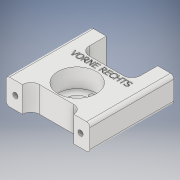
# Autodesk Inventor part: Motorhalterung leicht VR
Saved by Autodesk Inventor 2018 (Build 220112000, 112)
## iProperties
Created: 2019-03-03
Part Number: Motorhalterung leicht VR
Material: ABS-Kunststoff
Document SubType Name: Modeling
Designer: RedBots
Density: 0.513105 g/cm^3
Appearance: Weiß
Mass: 11 g
Surface Area: 84.958 cm^2
Volume: 21.4381 cm^3
Author: RedBots
Autodesk Inventor part; units mm, degrees
ref_plane "YZ Plane" through (0, 0, 0) normal (1, 0, 0) x (0, 1, 0)
ref_plane "XZ Plane" through (0, 0, 0) normal (0, 1, 0) x (-1, 0, 0)
ref_plane "XY Plane" through (0, 0, 0) normal (0, 0, 1) x (1, 0, 0)
sketch "Skizze2" plane through (0, 0, 0) normal (0, 0, 1) x (1, 0, 0)
  line L0 (0, 0) -> (49, 0)
  line L1 (0, 0) -> (49, 0) construction
  line L2 (49, 0) -> (49, 49)
  line L3 (49, 49) -> (0, 49)
  line L4 (0, 49) -> (0, 0)
  dimension "d16" = 49
  dimension "d18" = 49
  constraints: 10 end point, 2 equal length, 2 horizontal, 2 perpendicular
  measures "d16" distance of L0.start L0.end
  measures "d18" distance of L0.end L2.end
extrude "Extrusion1" add sketch "Skizze2" along normal blind 15
sketch "Skizze3" plane through (0, 0, 15) normal (0, 0, 1) x (1, 0, 0)
  circle A0 centre (24.5, 17) radius 11.25
  line L0 (0, 49) -> (0, 0) construction
  line L1 (0, 17) -> (49, 17) construction
  line L2 (49, 0) -> (49, 49) construction
  line L3 (0, 0) -> (49, 0) construction
  dimension "d72" = 22.5
  dimension "d73" = 17
  constraints: 2 end point, 2 point on line, 1 centre point, 1 coincident, 1 horizontal, 1 midpoint
  measures "d72" diameter of A0
  measures "d73" distance between parallel lines of L3 L1
extrude "Extrusion2" cut sketch "Skizze3" against normal blind 11
sketch "Skizze4" plane through (24.5, 17, 4) normal (0, 0, 1) x (1, 0, 0)
  circle A0 centre (7.3612, -4.25) radius 1.5
  circle A1 centre (0, 8.5) radius 1.5
  circle A2 centre (-7.3612, -4.25) radius 1.5
  line L0 (0, 0) -> (0, 8.5) construction
  line L1 (-24.5, -17) -> (24.5, -17) construction
  circle A3 centre (0, 0) radius 11.25 construction
  line L2 (0, -17) -> (0, 0) construction
  line L3 (0, 0) -> (7.3612, -4.25) construction
  line L4 (0, 0) -> (-7.3612, -4.25) construction
  circle A4 centre (0, 0) radius 6.5
  dimension "d37" = 3
  dimension "d42" = 3
  dimension "d43" = 3
  dimension "d90" = 8.5
  dimension "d91" = 120
  dimension "d92" = 120
  dimension "d93" = 13
  constraints: 8 end point, 4 centre point, 4 coincident, 2 equal length, 2 vertical, 1 midpoint
  measures "d37" diameter of A0
  measures "d42" diameter of A1
  measures "d43" diameter of A2
  measures "d90" distance of L0.start L0.end
  measures "d91" angle of L3 L0
  measures "d92" angle of L0 L4
  measures "d93" diameter of A4
extrude "Extrusion3" cut sketch "Skizze4" against normal up to next
sketch "Skizze9" plane through (0, 49, 0) normal (0, 1, 0) x (1, 0, 0)
  line L0 (24.5, -7.5) -> (43.5, -7.5) construction
  circle A0 centre (5.5, -7.5) radius 1.5
  circle A1 centre (43.5, -7.5) radius 1.5
  line L1 (0, -15) -> (49, -15) construction
  line L2 (24.5, -15) -> (24.5, 0) construction
  line L3 (49, 0) -> (0, 0) construction
  line L4 (5.5, -7.5) -> (24.5, -7.5) construction
  dimension "d58" = 3
  dimension "d89" = 19
  constraints: 7 end point, 3 midpoint, 2 centre point, 2 collinear, 1 coincident, 1 equal radius, 1 horizontal, 1 vertical
  measures "d58" diameter of A0
  measures "d89" distance of L0.start L0.end
extrude "Extrusion6" cut sketch "Skizze9" against normal blind 56
sketch "Skizze12" plane through (0, 0, 0) normal (0, 0, -1) x (-1, 0, 0)
  circle A0 centre (-24.5, 25.5) radius 1.5 projected
  circle A1 centre (-24.5, 25.5) radius 3
  circle A2 centre (-17.1388, 12.75) radius 1.5 projected
  circle A3 centre (-17.1388, 12.75) radius 3
  circle A4 centre (-31.8612, 12.75) radius 1.5 projected
  circle A5 centre (-31.8612, 12.75) radius 3
  point P0 (0, 0)
  dimension "d80" = 6
  dimension "d81" = 6
  dimension "d82" = 6
  constraints: 3 centre point, 3 coincident
  measures "d80" diameter of A1
  measures "d81" diameter of A3
  measures "d82" diameter of A5
extrude "Extrusion8" cut sketch "Skizze12" against normal blind 0.16
chamfer "Fase3" distance 1.5 angle 45 3 edges at (23, 25.5, 0.16) (30.3612, 12.75, 0.16) (15.6388, 12.75, 0.16)
fillet "Rundung2" radius 0.5 3 edges at (23, 25.5, 1.66) (30.3612, 12.75, 1.66) (15.6388, 12.75, 1.66)
sketch "Skizze14" plane through (0, 0, 0) normal (0, 0, -1) x (-1, 0, 0)
  line L0 (-39.5, 49) -> (-9.5, 49)
  line L1 (-9.5, 49) -> (-9.5, 34)
  line L2 (-9.5, 34) -> (-39.5, 34)
  line L3 (-39.5, 34) -> (-39.5, 49)
  line L4 (-49, 49) -> (0, 49) projected
  line L5 (-49, 0) -> (-49, 49) construction
  line L6 (0, 49) -> (0, 0) construction
  line L7 (-39.5, 0) -> (-9.5, 0)
  line L8 (-9.5, 0) -> (-9.5, 5)
  line L9 (-9.5, 5) -> (-39.5, 5)
  line L10 (-39.5, 5) -> (-39.5, 0)
  line L11 (0, 0) -> (-49, 0) projected
  point P0 (-24.5, 49)
  point P1 (-24.5, 0)
  point P2 (-24.5, 0)
  dimension "d95" = 15
  dimension "d96" = 30
  dimension "d101" = 5
  constraints: 16 end point, 6 midpoint, 3 horizontal, 3 parallel, 2 vertical, 1 perpendicular
  measures "d95" distance of L0.end L1.end
  measures "d96" distance between parallel lines of L1 L3
  measures "d101" distance of L7.end L9.start
extrude "Extrusion9" cut sketch "Skizze14" against normal up to next
fillet "Rundung3" radius 5 4 edges at (39.5, 34, 7.5) (9.5, 34, 7.5) (39.5, 5, 7.5) (9.5, 5, 7.5)
fillet "Rundung4" radius 2 4 edges at (49, 24.5, 15) (49, 24.5, 0) (0, 24.5, 0) (0, 24.5, 15)
sketch "Skizze15" plane through (0, 0, 15) normal (0, 0, 1) x (1, 0, 0)
  line L0 (14.5, 34) -> (34.5, 34) construction
  line L1 (24.5, 34) -> (24.5, 28.25) construction
  circle A0 centre (24.5, 17) radius 11.25 construction
  line L2 (10.3922, 32.875) -> (9.1868, 29.375)
  line L3 (9.1868, 29.375) -> (8.6848, 29.375)
  line L4 (8.6848, 29.375) -> (7.4793, 32.875)
  line L5 (7.4793, 32.875) -> (7.9785, 32.875)
  line L6 (7.9785, 32.875) -> (8.9485, 29.9678)
  line L7 (8.9485, 29.9678) -> (9.9186, 32.875)
  line L8 (9.9186, 32.875) -> (10.3922, 32.875)
  spline S0 degree 2 poles (13.203, 32.4751) (13.4015, 32.2425) (13.6228, 31.5618) (13.6228, 31.125) knots 0 0 0 1 2 2 2
  spline S1 degree 2 poles (13.6228, 31.125) (13.6228, 30.6996) (13.4072, 30.0103) (13.203, 29.7778) knots 0 0 0 1 2 2 2
  spline S2 degree 2 poles (13.203, 29.7778) (12.9874, 29.5338) (12.4173, 29.3013) (12.0741, 29.3013) knots 0 0 0 1 2 2 2
  spline S3 degree 2 poles (12.0741, 29.3013) (11.7196, 29.3013) (11.1523, 29.5423) (10.9453, 29.7778) knots 0 0 0 1 2 2 2
  spline S4 degree 2 poles (10.9453, 29.7778) (10.7439, 30.0103) (10.5284, 30.6939) (10.5284, 31.125) knots 0 0 0 1 2 2 2
  spline S5 degree 2 poles (10.5284, 31.125) (10.5284, 31.5646) (10.7468, 32.234) (10.9481, 32.4751) knots 0 0 0 1 2 2 2
  spline S6 degree 2 poles (10.9481, 32.4751) (11.1523, 32.7077) (11.7224, 32.9487) (12.0741, 32.9487) knots 0 0 0 1 2 2 2
  spline S7 degree 2 poles (12.0741, 32.9487) (12.4315, 32.9487) (13.0045, 32.6991) (13.203, 32.4751) knots 0 0 0 1 2 2 2
  spline S8 degree 2 poles (13.1378, 31.125) (13.1378, 31.471) (12.9874, 32.0071) (12.8513, 32.1829) knots 0 0 0 1 2 2 2
  spline S9 degree 2 poles (12.8513, 32.1829) (12.7123, 32.3645) (12.3209, 32.546) (12.077, 32.546) knots 0 0 0 1 2 2 2
  spline S10 degree 2 poles (12.077, 32.546) (11.8246, 32.546) (11.4445, 32.3701) (11.2998, 32.1829) knots 0 0 0 1 2 2 2
  spline S11 degree 2 poles (11.2998, 32.1829) (11.1609, 32.0043) (11.0134, 31.4654) (11.0134, 31.125) knots 0 0 0 1 2 2 2
  spline S12 degree 2 poles (11.0134, 31.125) (11.0134, 30.4358) (11.592, 29.704) (12.077, 29.704) knots 0 0 0 1 2 2 2
  spline S13 degree 2 poles (12.077, 29.704) (12.562, 29.704) (13.1378, 30.4358) (13.1378, 31.125) knots 0 0 0 1 2 2 2
  line L9 (16.842, 29.375) -> (16.2378, 29.375)
  line L10 (16.2378, 29.375) -> (15.1317, 30.7676)
  line L11 (15.1317, 30.7676) -> (14.5985, 30.7676)
  line L12 (14.5985, 30.7676) -> (14.5985, 29.375)
  line L13 (14.5985, 29.375) -> (14.1333, 29.375)
  line L14 (14.1333, 29.375) -> (14.1333, 32.875)
  line L15 (14.1333, 32.875) -> (15.0353, 32.875)
  spline S14 degree 2 poles (15.0353, 32.875) (15.3359, 32.875) (15.7415, 32.8098) (15.9259, 32.6906) knots 0 0 0 1 2 2 2
  spline S15 degree 2 poles (15.9259, 32.6906) (16.1102, 32.5715) (16.3229, 32.2) (16.3229, 31.9248) knots 0 0 0 1 2 2 2
  spline S16 degree 2 poles (16.3229, 31.9248) (16.3229, 31.5419) (15.9315, 31.0229) (15.5968, 30.8981) knots 0 0 0 1 2 2 2
  line L16 (15.5968, 30.8981) -> (16.842, 29.375)
  spline S17 degree 2 poles (15.8379, 31.888) (15.8379, 32.0411) (15.7301, 32.2765) (15.6167, 32.3531) knots 0 0 0 1 2 2 2
  spline S18 degree 2 poles (15.6167, 32.3531) (15.5174, 32.4184) (15.2536, 32.4722) (15.0608, 32.4722) knots 0 0 0 1 2 2 2
  line L17 (15.0608, 32.4722) -> (14.5985, 32.4722)
  line L18 (14.5985, 32.4722) -> (14.5985, 31.1562)
  line L19 (14.5985, 31.1562) -> (15.0069, 31.1562)
  spline S19 degree 2 poles (15.0069, 31.1562) (15.2083, 31.1562) (15.5288, 31.2271) (15.6394, 31.3377) knots 0 0 0 1 2 2 2
  spline S20 degree 2 poles (15.6394, 31.3377) (15.7415, 31.4342) (15.8379, 31.7064) (15.8379, 31.888) knots 0 0 0 1 2 2 2
  line L20 (19.6244, 29.375) -> (19.1025, 29.375)
  line L21 (19.1025, 29.375) -> (17.5539, 32.3928)
  line L22 (17.5539, 32.3928) -> (17.5539, 29.375)
  line L23 (17.5539, 29.375) -> (17.1199, 29.375)
  line L24 (17.1199, 29.375) -> (17.1199, 32.875)
  line L25 (17.1199, 32.875) -> (17.7808, 32.875)
  line L26 (17.7808, 32.875) -> (19.1904, 30.1039)
  line L27 (19.1904, 30.1039) -> (19.1904, 32.875)
  line L28 (19.1904, 32.875) -> (19.6244, 32.875)
  line L29 (19.6244, 32.875) -> (19.6244, 29.375)
  line L30 (20.3335, 29.375) -> (20.3335, 32.875)
  line L31 (20.3335, 32.875) -> (22.5231, 32.875)
  line L32 (22.5231, 32.875) -> (22.5231, 32.4609)
  line L33 (22.5231, 32.4609) -> (20.7986, 32.4609)
  line L34 (20.7986, 32.4609) -> (20.7986, 31.5022)
  line L35 (20.7986, 31.5022) -> (22.4068, 31.5022)
  line L36 (22.4068, 31.5022) -> (22.4068, 31.0881)
  line L37 (22.4068, 31.0881) -> (20.7986, 31.0881)
  line L38 (20.7986, 31.0881) -> (20.7986, 29.7891)
  line L39 (20.7986, 29.7891) -> (22.5231, 29.7891)
  line L40 (22.5231, 29.7891) -> (22.5231, 29.375)
  line L41 (22.5231, 29.375) -> (20.3335, 29.375)
  line L42 (27.2455, 29.375) -> (26.6414, 29.375)
  line L43 (26.6414, 29.375) -> (25.5353, 30.7676)
  line L44 (25.5353, 30.7676) -> (25.002, 30.7676)
  line L45 (25.002, 30.7676) -> (25.002, 29.375)
  line L46 (25.002, 29.375) -> (24.5369, 29.375)
  line L47 (24.5369, 29.375) -> (24.5369, 32.875)
  line L48 (24.5369, 32.875) -> (25.4388, 32.875)
  spline S21 degree 2 poles (25.4388, 32.875) (25.7395, 32.875) (26.1451, 32.8098) (26.3294, 32.6906) knots 0 0 0 1 2 2 2
  spline S22 degree 2 poles (26.3294, 32.6906) (26.5138, 32.5715) (26.7265, 32.2) (26.7265, 31.9248) knots 0 0 0 1 2 2 2
  spline S23 degree 2 poles (26.7265, 31.9248) (26.7265, 31.5419) (26.3351, 31.0229) (26.0004, 30.8981) knots 0 0 0 1 2 2 2
  line L49 (26.0004, 30.8981) -> (27.2455, 29.375)
  spline S24 degree 2 poles (26.2415, 31.888) (26.2415, 32.0411) (26.1337, 32.2765) (26.0203, 32.3531) knots 0 0 0 1 2 2 2
  spline S25 degree 2 poles (26.0203, 32.3531) (25.921, 32.4184) (25.6572, 32.4722) (25.4643, 32.4722) knots 0 0 0 1 2 2 2
  line L50 (25.4643, 32.4722) -> (25.002, 32.4722)
  line L51 (25.002, 32.4722) -> (25.002, 31.1562)
  line L52 (25.002, 31.1562) -> (25.4105, 31.1562)
  spline S26 degree 2 poles (25.4105, 31.1562) (25.6118, 31.1562) (25.9323, 31.2271) (26.0429, 31.3377) knots 0 0 0 1 2 2 2
  spline S27 degree 2 poles (26.0429, 31.3377) (26.1451, 31.4342) (26.2415, 31.7064) (26.2415, 31.888) knots 0 0 0 1 2 2 2
  line L53 (27.5235, 29.375) -> (27.5235, 32.875)
  line L54 (27.5235, 32.875) -> (29.7131, 32.875)
  line L55 (29.7131, 32.875) -> (29.7131, 32.4609)
  line L56 (29.7131, 32.4609) -> (27.9887, 32.4609)
  line L57 (27.9887, 32.4609) -> (27.9887, 31.5022)
  line L58 (27.9887, 31.5022) -> (29.5968, 31.5022)
  line L59 (29.5968, 31.5022) -> (29.5968, 31.0881)
  line L60 (29.5968, 31.0881) -> (27.9887, 31.0881)
  line L61 (27.9887, 31.0881) -> (27.9887, 29.7891)
  line L62 (27.9887, 29.7891) -> (29.7131, 29.7891)
  line L63 (29.7131, 29.7891) -> (29.7131, 29.375)
  line L64 (29.7131, 29.375) -> (27.5235, 29.375)
  spline S28 degree 2 poles (31.5908, 29.3126) (31.2504, 29.3126) (30.6746, 29.5423) (30.4647, 29.7721) knots 0 0 0 1 2 2 2
  spline S29 degree 2 poles (30.4647, 29.7721) (30.2549, 29.999) (30.0251, 30.6797) (30.0251, 31.1222) knots 0 0 0 1 2 2 2
  spline S30 degree 2 poles (30.0251, 31.1222) (30.0251, 31.5618) (30.2492, 32.2141) (30.4619, 32.4552) knots 0 0 0 1 2 2 2
  spline S31 degree 2 poles (30.4619, 32.4552) (30.6718, 32.6906) (31.2447, 32.9374) (31.5993, 32.9374) knots 0 0 0 1 2 2 2
  spline S32 degree 2 poles (31.5993, 32.9374) (31.7751, 32.9374) (32.0843, 32.8863) (32.2147, 32.8466) knots 0 0 0 1 2 2 2
  spline S33 degree 2 poles (32.2147, 32.8466) (32.3282, 32.8098) (32.5636, 32.7048) (32.6799, 32.6424) knots 0 0 0 1 2 2 2
  line L65 (32.6799, 32.6424) -> (32.6799, 32.0808)
  line L66 (32.6799, 32.0808) -> (32.643, 32.0808)
  spline S34 degree 2 poles (32.643, 32.0808) (32.5806, 32.1376) (32.3878, 32.2964) (32.2488, 32.373) knots 0 0 0 1 2 2 2
  spline S35 degree 2 poles (32.2488, 32.373) (32.1155, 32.4467) (31.8006, 32.5403) (31.5964, 32.5403) knots 0 0 0 1 2 2 2
  spline S36 degree 2 poles (31.5964, 32.5403) (31.3724, 32.5403) (30.9724, 32.356) (30.8221, 32.1801) knots 0 0 0 1 2 2 2
  spline S37 degree 2 poles (30.8221, 32.1801) (30.6746, 32.0014) (30.5101, 31.4597) (30.5101, 31.1222) knots 0 0 0 1 2 2 2
  spline S38 degree 2 poles (30.5101, 31.1222) (30.5101, 30.762) (30.6831, 30.2429) (30.8335, 30.0642) knots 0 0 0 1 2 2 2
  spline S39 degree 2 poles (30.8335, 30.0642) (30.981, 29.8912) (31.3752, 29.7154) (31.5964, 29.7154) knots 0 0 0 1 2 2 2
  spline S40 degree 2 poles (31.5964, 29.7154) (31.7978, 29.7154) (32.141, 29.8146) (32.2743, 29.8884) knots 0 0 0 1 2 2 2
  spline S41 degree 2 poles (32.2743, 29.8884) (32.4019, 29.9621) (32.592, 30.1153) (32.6459, 30.1692) knots 0 0 0 1 2 2 2
  line L67 (32.6459, 30.1692) -> (32.6799, 30.1692)
  line L68 (32.6799, 30.1692) -> (32.6799, 29.6132)
  spline S42 degree 2 poles (32.6799, 29.6132) (32.5636, 29.5594) (32.3594, 29.4601) (32.2147, 29.4147) knots 0 0 0 1 2 2 2
  spline S43 degree 2 poles (32.2147, 29.4147) (32.0616, 29.3637) (31.8006, 29.3126) (31.5908, 29.3126) knots 0 0 0 1 2 2 2
  line L69 (35.6552, 29.375) -> (35.19, 29.375)
  line L70 (35.19, 29.375) -> (35.19, 31.0881)
  line L71 (35.19, 31.0881) -> (33.579, 31.0881)
  line L72 (33.579, 31.0881) -> (33.579, 29.375)
  line L73 (33.579, 29.375) -> (33.1139, 29.375)
  line L74 (33.1139, 29.375) -> (33.1139, 32.875)
  line L75 (33.1139, 32.875) -> (33.579, 32.875)
  line L76 (33.579, 32.875) -> (33.579, 31.5022)
  line L77 (33.579, 31.5022) -> (35.19, 31.5022)
  line L78 (35.19, 31.5022) -> (35.19, 32.875)
  line L79 (35.19, 32.875) -> (35.6552, 32.875)
  line L80 (35.6552, 32.875) -> (35.6552, 29.375)
  line L81 (37.1811, 29.375) -> (37.1811, 32.4609)
  line L82 (37.1811, 32.4609) -> (36.0069, 32.4609)
  line L83 (36.0069, 32.4609) -> (36.0069, 32.875)
  line L84 (36.0069, 32.875) -> (38.8205, 32.875)
  line L85 (38.8205, 32.875) -> (38.8205, 32.4609)
  line L86 (38.8205, 32.4609) -> (37.6463, 32.4609)
  line L87 (37.6463, 32.4609) -> (37.6463, 29.375)
  line L88 (37.6463, 29.375) -> (37.1811, 29.375)
  spline S44 degree 2 poles (40.1507, 29.3126) (39.7707, 29.3126) (39.2374, 29.4714) (39.002, 29.5849) knots 0 0 0 1 2 2 2
  line L89 (39.002, 29.5849) -> (39.002, 30.1692)
  line L90 (39.002, 30.1692) -> (39.0361, 30.1692)
  spline S45 degree 2 poles (39.0361, 30.1692) (39.2658, 29.9536) (39.8472, 29.7154) (40.1167, 29.7154) knots 0 0 0 1 2 2 2
  spline S46 degree 2 poles (40.1167, 29.7154) (40.5024, 29.7154) (40.8967, 30.0359) (40.8967, 30.2996) knots 0 0 0 1 2 2 2
  spline S47 degree 2 poles (40.8967, 30.2996) (40.8967, 30.5095) (40.6896, 30.7705) (40.4656, 30.8357) knots 0 0 0 1 2 2 2
  spline S48 degree 2 poles (40.4656, 30.8357) (40.3039, 30.8811) (40.0344, 30.9435) (39.8331, 30.9945) knots 0 0 0 1 2 2 2
  spline S49 degree 2 poles (39.8331, 30.9945) (39.6515, 31.0427) (39.3651, 31.1874) (39.2545, 31.3037) knots 0 0 0 1 2 2 2
  spline S50 degree 2 poles (39.2545, 31.3037) (39.1467, 31.42) (39.0276, 31.732) (39.0276, 31.9362) knots 0 0 0 1 2 2 2
  spline S51 degree 2 poles (39.0276, 31.9362) (39.0276, 32.3616) (39.6912, 32.9374) (40.2046, 32.9374) knots 0 0 0 1 2 2 2
  spline S52 degree 2 poles (40.2046, 32.9374) (40.4996, 32.9374) (41.0215, 32.8211) (41.2455, 32.7105) knots 0 0 0 1 2 2 2
  line L91 (41.2455, 32.7105) -> (41.2455, 32.1546)
  line L92 (41.2455, 32.1546) -> (41.2115, 32.1546)
  spline S53 degree 2 poles (41.2115, 32.1546) (41.0442, 32.3077) (40.5223, 32.5346) (40.2358, 32.5346) knots 0 0 0 1 2 2 2
  spline S54 degree 2 poles (40.2358, 32.5346) (39.9125, 32.5346) (39.5126, 32.2312) (39.5126, 31.9844) knots 0 0 0 1 2 2 2
  spline S55 degree 2 poles (39.5126, 31.9844) (39.5126, 31.7632) (39.748, 31.4994) (39.9692, 31.4398) knots 0 0 0 1 2 2 2
  spline S56 degree 2 poles (39.9692, 31.4398) (40.1167, 31.4001) (40.545, 31.298) (40.6868, 31.2555) knots 0 0 0 1 2 2 2
  spline S57 degree 2 poles (40.6868, 31.2555) (41.047, 31.1449) (41.3817, 30.6996) (41.3817, 30.3734) knots 0 0 0 1 2 2 2
  spline S58 degree 2 poles (41.3817, 30.3734) (41.3817, 30.1663) (41.2143, 29.7692) (41.064, 29.6303) knots 0 0 0 1 2 2 2
  spline S59 degree 2 poles (41.064, 29.6303) (40.8967, 29.4771) (40.4712, 29.3126) (40.1507, 29.3126) knots 0 0 0 1 2 2 2
  point P0 (0, 0)
  point P1 (24.5, 31.125)
  point P2 (24.5, 31.125)
  constraints: 2 end point, 2 midpoint, 1 coincident, 1 vertical, 1 vertical alignment, 2 other
emboss "Prägen1" sketch "Skizze15" operation cut depth 1 direction (0, 0, -1)
